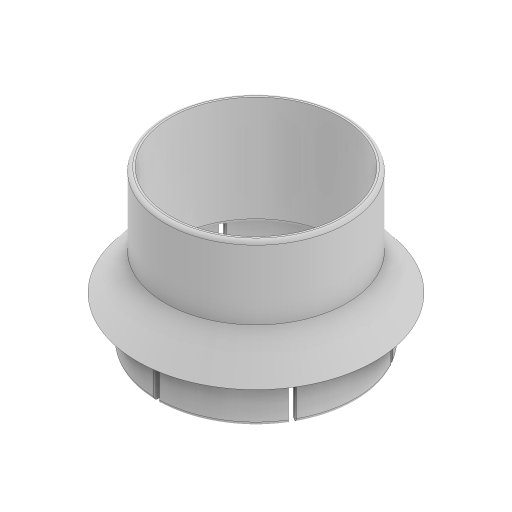
# Autodesk Inventor part: top-ventilation-tube-adapter-109.6mmID-to-100mmID
Saved by Autodesk Inventor 2023 (Build 270158000, 158)
## iProperties
Created: 2024-07-10
Part Number: top-ventilation-tube-adapter-109.6mmID-to-100mmID
Material: Generic
Document SubType Name: Modeling
Designer: N.Vladimirov
Density: 1 g/cm^3
Appearance: Default
Author: N.Vladimirov
Autodesk Inventor part; units mm, degrees
ref_plane "YZ Plane" through (0, 0, 0) normal (1, 0, 0) x (0, 1, 0)
ref_plane "XZ Plane" through (0, 0, 0) normal (0, 1, 0) x (-1, 0, 0)
ref_plane "XY Plane" through (0, 0, 0) normal (0, 0, 1) x (1, 0, 0)
sketch "Sketch1" plane through (0, 0, 0) normal (0, 0, 1) x (1, 0, 0)
  line L0 (-54.7, 0) -> (-49, 0)
  line L1 (-50.7, -25) -> (-52.7, -25)
  line L2 (-54.7, -23) -> (-54.7, 0)
  line L3 (-47, 20) -> (-50, 20)
  line L4 (-50, 20) -> (-50, 58)
  line L5 (-48, 60) -> (-47, 60)
  line L6 (-47, 60) -> (-47, 20)
  line L7 (-54.7, 0) -> (-65.3724, 0)
  line L8 (-65.3724, 0) -> (-50, 20)
  line L9 (-47, 20) -> (-47, 2)
  arc A0 (-48, 60) -> (-50, 58) centre (-48, 58) ccw
  arc A1 (-54.7, -23) -> (-52.7, -25) centre (-52.7, -23) ccw
  line L10 (0, -42.5799) -> (0, 77.5799) projected
  line L11 (-50.7, -25) -> (-50.7, 0)
  arc A2 (-49, 0) -> (-47, 2) centre (-49, 2) ccw
  point P0 (0, 0)
  point P1 (-47, 0)
  point P2 (-54.7, -25)
  point P3 (-50, 60)
  point P4 (-51.85, 0)
  dimension "d7" = 40
  dimension "d10" = 2
  dimension "d12" = 20
  dimension "d20" = 50
  dimension "d21" = 54.7
  dimension "d22" = 3
  dimension "d23" = 2
  dimension "d24" = 4
  constraints: 22 end point, 7 point on line, 6 point on circle, 6 tangent, 3 centre point, 3 horizontal, 3 parallel, 2 perpendicular, 1 equal radius, 1 midpoint, 1 vertical
  measures "d7" distance of L3.end point (-50, 60)
  measures "d10" radius of A0
  measures "d12" distance from line of point (-51.85, 0) L3
  measures "d20" distance between parallel lines of L10 L4
  measures "d21" distance between parallel lines of L10 L2
  measures "d22" distance between parallel lines of L4 L6
  measures "d23" radius of A2
  measures "d24" distance between parallel lines of L2 L11
revolve "Revolution1" add sketch "Sketch1" angle 360 about axis through (0, -10, 0) along (0, 1, 0)
sketch "Sketch2" plane through (0, -25, 0) normal (0, -1, 0) x (1, 0, 0)
  line L0 (1.5, 45.7) -> (-1.5, 45.7)
  line L1 (-1.5, 45.7) -> (-1.5, 55.7)
  line L2 (-1.5, 55.7) -> (1.5, 55.7)
  line L3 (1.5, 55.7) -> (1.5, 45.7)
  circle A0 centre (0, 0) radius 50.7 projected
  line L4 (1.5, 45.7) -> (-1.5, 55.7) construction
  line L5 (-1.5, 45.7) -> (1.5, 55.7) construction
  point P0 (0, 50.7)
  dimension "d13" = 3
  dimension "d14" = 10
  constraints: 12 end point, 2 midpoint, 2 parallel, 1 horizontal, 1 perpendicular, 1 vertical alignment, 1 other
  measures "d13" distance of L1.end L2.end
  measures "d14" distance of L0.end L1.end
extrude "Extrusion1" cut sketch "Sketch2" against normal blind 25 contours L0 L1 A0 L3 | A0 L1 L2 L3 picked at (0.1667, 47.3658)
pattern_circular "Circular Pattern1" count 6 over 360 about axis through (0, -10, 0) along (0, 1, 0) of "Extrusion1"
body "Solid1"
